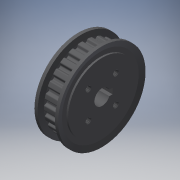
# Autodesk Inventor part: ATP25XL025-A-N8-KC90-QFC20-M3-FC45.0-TPC3_b
Saved by Autodesk Inventor 2017 (Build 210142000, 142)
## iProperties
Category: PARTsolutions
Company: MISUMI
Created: 2017-08-07
Part Number: ATP25XL025-A-N8-KC90-QFC20-M3-FC45.0-TPC3_b
Catalog Web Link: www.cadenas.de
Description: ATP__XL025, ATP__XL031, ATP__ XL037, ATP__XL050, BTP__XL025, BTP__XL031, BTP__XL037, BTP__XL050, KTP__XL025, KTP__XL031, KTP__ XL037, KTP__XL050, NTP__XL025, NTP__XL031, NTP__ XL037, NTP__XL050, MTP__XL025, MTP__ XL037, MTP__XL050, MTPB__XL025, MTPB__ XL037, MTPB__XL050, MTPP__XL025, MTPP__ XL037, MTPP__XL050, STP__XL025, STP__ XL037, STP__XL050_body-Timing Pulleys XL Type
Vendor: MISUMI
Document SubType Name: Modeling
Designer: psAdmin
Manufacturer: MISUMI
Mass: 14.7534 g
Surface Area: 66.1707 cm^2
Volume: 14.7534 cm^3
Density: 1 g/cm^3
Material: 일반
Appearance: PSOLRGB-192-192-192
PSOL_IDENT_0: {$CADENAS_DATA\23d-libs\misumi\metric\51_timing_pulleys\mtp_xl\mtp_xl.prj},737 {VTYP=3D},{NB=ATP25XL
PSOL_IDENT_1: 025-A-N8-KC90-QFC20-M3-FC45.0-TPC3_b},{LINA=ATP25XL025-A-N8-KC90-QFC20-M3-FC45.0-TPC3},{NN=ATP__XL02
PSOL_IDENT_2: 5, ATP__XL031, ATP__ XL037, ATP__XL050, BTP__XL025, BTP__XL031, BTP__XL037, BTP__XL050, KTP__XL025,
PSOL_IDENT_3: KTP__XL031, KTP__ XL037, KTP__XL050, NTP__XL025, NTP__XL031, NTP__ XL037, NTP__XL050, MTP__XL025, MT
PSOL_IDENT_4: P__ XL037, MTP__XL050, MTPB__XL025, MTPB__ XL037, MTPB__XL050, MTPP__XL025, MTPP__ XL037, MTPP__XL05
PSOL_IDENT_5: 0, STP__XL025, STP__ XL037, STP__XL050_body},{DATE=27.04.2017 02:25:46},{GEOMDATE=02.12.2016 00:36:0
PSOL_IDENT_6: 0},{VERSION=},{LINEID=120},{LINESUBID=-1},{WBVAR=MATP,ST,TNW,PS,SBS,DD,Z,J,Q,R,S,T,ALT1,ALT2,M,QSC,Q
PSOL_IDENT_7: FC,QTC,ALT3,K,KSC,KFC,KTC,ALT4,ZM,ZSC,ZFC,ZTC,ALT5,ALT6,ALT7,FC,ALT8,SRG,ALT9,BTC,TL,ALT10,TPC,ALT11
PSOL_IDENT_8: ,BC,ALT12,SLH}  {NB=ATP25XL025-A-N8-KC90-QFC20-M3-FC45.0-TPC3_b},{LINA=ATP25XL025-A-N8-KC90-QFC20-M3
PSOL_IDENT_9: -FC45.0-TPC3},{KT=DUMMY},{PN=ATP25XL025-A-N8-KC90-QFC20-M3-FC45.0-TPC3},{TYPE=ATP},{MATP=A2017},{MAT
PSOL_IDENT_10: PALG= 'A2017','Aluminum Alloy 2000 series','S45C','1045 Carbon Steel Equivalent','SUS304','SUS304' }
PSOL_IDENT_11: ,{ST=CA},{STALG= 'CA','Clear Anodize','BA','Black Anodize','HAT','Hard Clear Anodize','ENP','Electro
PSOL_IDENT_12: less Nickel Plating' },{NT=25},{TNW=XL025},{TNWALG= 'XL025','XL031','XL037','XL050' },{BW=6.4mm (1/4
PSOL_IDENT_13: inch)},{PS=A},{PSALG= 'A','B' },{SBS=N},{SBSALG= 'H','Round Hole','P','Round Hole + Tap','N','New JI
PSOL_IDENT_14: S Keywayed Bore + Tap (Standard)','NK','New JIS Keywayed Bore + Tap (width 4.0mm, height 1.8mm)','C'
PSOL_IDENT_15: ,'Old JIS Keywayed Bore + Tap','V','Stepped Hole','Y','Both Ends Stepped Hole','WB','Double Stepped
PSOL_IDENT_16: Hole' },{DD=8.00},{DDALG=[8:8/1],[10:22/1]},{DDHA=[8:12/1],12.7,[13:31/1]},{DDPA=[8:12/1],12.7,[13:2
PSOL_IDENT_17: 5/1]},{DDNA=[8:8/1],[10:22/1]},{DDNK=[10:10/1]},{DDCA=[10,12,15,16,18,19,20]},{DDVA=[8:12/1],12.7,[1
PSOL_IDENT_18: 3:29/1]},{DDY=[8:29/1]},{DDWB=[8:27/1]},{DDHB=},{DDPB=},{DDNB=},{DDCB=},{DDVFB=},{Z=0},{ZALG=[0]},{Z
PSOL_IDENT_19: MIN=10.000},{ZAMAX=31.000},{ZBMAX=0.000},{DDZ=8.000},{J=0.0},{JALG=[0]},{JMIN=2.000},{JMAX=10},{JPN=
PSOL_IDENT_20: },{Q=0},{QALG=[0]},{QRMIN=10.000},{QRMAX=31},{WBQMIN=12.000},{R=0},{RALG=[0]},{WBRMAX=-2.000},{S=0.0
PSOL_IDENT_21: },{SALG=[0]},{SMAX=6.5},{T=0.0},{TALG=[0]},{TMAX=8},{SBSPN=-N8},{A=7.5},{W=12.5},{L=0},{PD=40.43},{O
PSOL_IDENT_22: D=39.92},{D=0},{DALG=30.000},{DE=35},{F=48},{E=35},{TT=1.6},{BBK=3.000},{TTK=1.4},{ALT1=KC90},{ALT1A
PSOL_IDENT_23: LG= '','w/o KC90 (Set Screw Angle)','KC90','with KC90 (Set Screw Angle)' },{ANG=86.400},{ALT1PN=-KC9
PSOL_IDENT_24: 0},{ALT2=QFC},{ALT2ALG= '','w/o Side Tapped Hole','QFC','with QFC (4 Places Side Tapped Hole)' },{M=
PSOL_IDENT_25: M3},{MALG= 'M3','M4','M5','M6','M8' },{MFTALG= 'M3','M4','M5','M6','M8' },{MSALG='M3','M4','M5','M6'
PSOL_IDENT_26: ,'M8' },{M3D=3.000},{KDML=9.500},{ML=9.500},{MUL=0.500},{PITCH=0.500},{QSC=0.0},{QSCALG=0},{QFC=20.0
PSOL_IDENT_27: },{QFCALG=[15:28/0.5]},{QTC=0.0},{QTCALG=0},{QPCDMIN=15.000},{QPCDMINALG=15.000},{QPCDMAX=28.000},{A
PSOL_IDENT_28: LT2PN=-QFC20-M3},{TAP=6.000},{ALT3=},{ALT3ALG= '','Not applicable' },{K=0.0},{KALG=0},{KMIN=4.000},{
PSOL_IDENT_29: KFTMAX=9.500},{KSMAX=9.000},{KSC=0.0},{KSCALG=0},{KFC=0.0},{KFCALG=0},{KTC=0.0},{KTCALG=0},{KSCMIN=1
PSOL_IDENT_30: 2.000},{KPCDMIN=12.000},{KPCDMAX=31.000},{ALT3PN=},{ALT4=},{ALT4ALG= '','Not applicable' },{ALT4MIN=
PSOL_IDENT_31: 18.500},{ALT4MAX=24.500},{ZM=N/A},{ZMALG= 'N/A' },{ZMFTALG= 'N/A' },{ZMSALG= 'N/A' },{ZMDD1=0.0},{ZM
PSOL_IDENT_32: DD2=0.0},{ZMHH=0.0},{ZSC=0.0},{ZSCALG=[0]},{ZFC=0.0},{ZFCALG=[0]},{ZTC=0.0},{ZTCALG=[0]},{ZPCDMIN=0.
PSOL_IDENT_33: 000},{ZPCDMINALG=0.000},{ZPCDMAX=31.000},{ALT4PN=},{ALT5=},{ALT5ALG= '','w/o Flange not Attached','N
PSOL_IDENT_34: FC','with NFC (Flange not Attached)' },{ALT5PN=},{ALT6=},{ALT6ALG= '','w/o Flange Attached on One Si
PSOL_IDENT_35: de Only','RFC','with RFC (Flange Attached on The Boss Side Only)','LFC','with LFC (Flange Attached o
PSOL_IDENT_36: n The Opposite Side Only)' },{ALT6PN=},{ALT7=FC},{ALT7ALG= '','w/o FC (Flange Cut)','FC','with FC (F
PSOL_IDENT_37: lange Cut)' },{FC=45.0},{FCALG=[41:46/0.5]},{FCMIN=41.0},{FCMAX=46.0},{ALT7PN=-FC45.0},{ALT8=},{ALT8
PSOL_IDENT_38: ALG= '','Not applicable' },{ALT8ALGALG=13.000},{ALT8DD2=0.000},{ALT8MM=0.000},{ALT8NN=0.000},{QC=20.
PSOL_IDENT_39: 000},{KC=0.000},{ZC=0.000},{SRG=0.0},{SRGALG=[0]},{SRGMAX=0.000},{DD2=0.0},{MM=0.00},{NN=0.00},{ALT8
PSOL_IDENT_40: PN=},{ALT9=},{ALT9ALG= '','Not applicable' },{BTC9=9.000},{TL9=1.000},{BTC=0},{BTCALG=[0]},{TL=0.0},
PSOL_IDENT_41: {TLALG=0},{TLMIN=1.000},{TLMAX=-13.000},{BTCL=0},{BTCD=0},{ALT9PN=},{WLBCTL=12.500},{ALT10=TPC},{ALT
PSOL_IDENT_42: 10ALG= '','w/o TPC (Tapped Hole Dimension)','TPC','with TPC (Tapped Hole Dimension)' },{TPC=M3},{TPC
PSOL_IDENT_43: ALG= 'M3','M5' },{TPCM=4.000},{ALT10PN=-TPC3},{ALT11=},{ALT11ALG= '','Not applicable' },{BC=0.0},{BC
PSOL_IDENT_44: ALG=0},{BCMIN=6},{BCMAX=-13},{M1WBC=6.25},{ALT11PN=},{KTT=14.56},{ALT12=},{ALT12ALG= '','w/o SLH (Se
PSOL_IDENT_45: t Screw Length)','SLH','with SLH (Set Screw Length)' },{SLH=0},{SLHALG=[0]},{ALT12PN=},{AC=M3x3},{M1=
PSOL_IDENT_46: 3.000},{M1L=3.000},{KEYA=1.000},{KEYB=0.000},{KEYM=1.000}
NN: 0.00
NT: 25
NB: ATP25XL025-A-N8-KC90-QFC20-M3-FC45.0-TPC3_b
NBSYN: $PN._b
LINA: ATP25XL025-A-N8-KC90-QFC20-M3-FC45.0-TPC3
PN: ATP25XL025-A-N8-KC90-QFC20-M3-FC45.0-TPC3
MATP: Aluminum Alloy 2000 series
ST: Clear Anodize
TNW: XL025
BW: 6.4mm (1/4inch)
PS: A
SBS: New JIS Keywayed Bore + Tap (Standard)
DD: 8.00
Z: 0
J: 0.0
Q: 0
R: 0
S: 0.0
T: 0.0
A: 7.5
W: 12.5
L: 0
PD: 40.43
OD: 39.92
D: 0
F: 48
E: 35
TT: 1.6
ALT1: with KC90 (Set Screw Angle)
ALT2: with QFC (4 Places Side Tapped Hole)
M: M3
QSC: 0.0
QFC: 20.0
QTC: 0.0
ALT3: Not applicable
K: 0.0
KSC: 0.0
KFC: 0.0
KTC: 0.0
ALT4: Not applicable
ZM: N/A
ZMDD1: 0.0
ZMDD2: 0.0
ZMHH: 0.0
ZSC: 0.0
ZFC: 0.0
ZTC: 0.0
ALT5: w/o Flange not Attached
ALT6: w/o Flange Attached on One Side Only
ALT7: with FC (Flange Cut)
FC: 45.0
ALT8: Not applicable
SRG: 0.0
DD2: 0.0
MM: 0.00
ALT9: Not applicable
BTC: 0
TL: 0.0
BTCL: 0
BTCD: 0
ALT10: with TPC (Tapped Hole Dimension)
TPC: M3
ALT11: Not applicable
BC: 0.0
ALT12: w/o SLH (Set Screw Length)
SLH: 0
AC: M3x3
SUPPLIER: MISUMI
ARTICLENO: ATP25XL025-A-N8-KC90-QFC20-M3-FC45.0-TPC3_b
BOMINFO: ATP25XL025-A-N8-KC90-QFC20-M3-FC45.0-TPC3
CREATOR: CADENAS GmbH
Title: ATP25XL025-A-N8-KC90-QFC20-M3-FC45.0-TPC3
Author: Cadenas PARTsolutions
Comments: Timing Pulleys XL Type
Autodesk Inventor part; units mm, degrees
sketch "_____2" plane through (0, 0, 0) normal (0, 0, 1) x (1, 0, 0)
  line L0 (12.5, 0) -> (0, 0)
  line L1 (0, 0) -> (0, 17.5)
  line L2 (0, 17.5) -> (0.9, 17.5)
  line L3 (0.9, 17.5) -> (0.9, 19.749356)
  line L4 (0.9, 19.749356) -> (-0.127996, 23.58589)
  line L5 (-0.127996, 23.58589) -> (1.417485, 24)
  line L6 (1.417485, 24) -> (2.5, 19.96)
  line L7 (2.5, 19.96) -> (10, 19.96)
  line L8 (10, 19.96) -> (11.082515, 24)
  line L9 (11.082515, 24) -> (12.627996, 23.58589)
  line L10 (12.627996, 23.58589) -> (11.6, 19.749356)
  line L11 (11.6, 19.749356) -> (11.6, 17.5)
  line L12 (11.6, 17.5) -> (12.5, 17.5)
  line L13 (12.5, 17.5) -> (12.5, 0)
  line L14 (12.5, 0) -> (0, 0)
  constraints: 30 end point
revolve "Revolution1" add sketch "_____2" angle 360 about axis through (12.5, 0, 0) along (1, 0, 0)
sketch "Sketch2" plane through (12.5, 0, 0) normal (1, 0, 0) x (0, 0, -1)
  point P0 (0, 0)
hole "Hole1" at (12.5, 0, 0) direction (-1, 0, 0) diameter 8 depth 12.5
sketch "_____6" plane through (2.5, 0, 0) normal (1, 0, 0) x (0, 0, -1)
  arc A0 (-19.856937, 3.787913) -> (-20.17511, -1.26931) centre (0, 0) ccw
  arc A1 (-20.17511, -1.26931) -> (-19.225607, -6.246779) centre (0, 0) ccw
  arc A2 (-19.225607, -6.246779) -> (-17.068089, -10.831739) centre (0, 0) ccw
  arc A3 (-17.068089, -10.831739) -> (-13.83812, -14.736101) centre (0, 0) ccw
  arc A4 (-13.83812, -14.736101) -> (-9.738651, -17.71454) centre (0, 0) ccw
  arc A5 (-9.738651, -17.71454) -> (-5.027266, -19.579909) centre (0, 0) ccw
  arc A6 (-5.027266, -19.579909) -> (0, -20.215) centre (0, 0) ccw
  arc A7 (0, -20.215) -> (5.027266, -19.579909) centre (0, 0) ccw
  arc A8 (5.027266, -19.579909) -> (9.738651, -17.71454) centre (0, 0) ccw
  arc A9 (9.738651, -17.71454) -> (13.83812, -14.736101) centre (0, 0) ccw
  arc A10 (13.83812, -14.736101) -> (17.068089, -10.831739) centre (0, 0) ccw
  arc A11 (17.068089, -10.831739) -> (19.225607, -6.246779) centre (0, 0) ccw
  arc A12 (19.225607, -6.246779) -> (20.17511, -1.26931) centre (0, 0) ccw
  arc A13 (20.17511, -1.26931) -> (19.856937, 3.787913) centre (0, 0) ccw
  arc A14 (19.856937, 3.787913) -> (18.291079, 8.607128) centre (0, 0) ccw
  arc A15 (18.291079, 8.607128) -> (15.575925, 12.885526) centre (0, 0) ccw
  arc A16 (15.575925, 12.885526) -> (11.882079, 16.354279) centre (0, 0) ccw
  arc A17 (11.882079, 16.354279) -> (7.441638, 18.795432) centre (0, 0) ccw
  arc A18 (7.441638, 18.795432) -> (2.533611, 20.055599) centre (0, 0) ccw
  arc A19 (2.533611, 20.055599) -> (-2.533611, 20.055599) centre (0, 0) ccw
  arc A20 (-2.533611, 20.055599) -> (-7.441638, 18.795432) centre (0, 0) ccw
  arc A21 (-7.441638, 18.795432) -> (-11.882079, 16.354279) centre (0, 0) ccw
  arc A22 (-11.882079, 16.354279) -> (-15.575925, 12.885526) centre (0, 0) ccw
  arc A23 (-15.575925, 12.885526) -> (-18.291079, 8.607128) centre (0, 0) ccw
  arc A24 (-18.291079, 8.607128) -> (-19.856937, 3.787913) centre (0, 0) ccw
  arc A25 (-19.567688, 0.133077) -> (-19.954959, -0.448576) centre (-19.345113, -0.434867) ccw
  arc A26 (-19.954959, -0.448576) -> (-19.920613, -1.253299) centre (0, 0) ccw
  arc A27 (-19.920613, -1.253299) -> (-19.853829, -2.055981) centre (0, 0) ccw
  arc A28 (-19.853829, -2.055981) -> (-19.396712, -2.58451) centre (-19.247074, -1.993148) ccw
  line L0 (-19.396712, -2.58451) -> (-18.726173, -2.754182)
  arc A29 (-18.275172, -3.239087) -> (-18.726173, -2.754182) centre (-18.875811, -3.345543) ccw
  arc A30 (-18.275172, -3.239087) -> (-18.184213, -3.715914) centre (0, 0) ccw
  arc A31 (-18.425038, -4.332791) -> (-18.184213, -3.715914) centre (-18.781862, -3.838042) ccw
  line L1 (-18.425038, -4.332791) -> (-18.986028, -4.73739)
  arc A32 (-18.986028, -4.73739) -> (-19.216481, -5.397079) centre (-18.629204, -5.232139) ccw
  arc A33 (-19.216481, -5.397079) -> (-18.983088, -6.167979) centre (0, 0) ccw
  arc A34 (-18.983088, -6.167979) -> (-18.718783, -6.928835) centre (0, 0) ccw
  arc A35 (-18.718783, -6.928835) -> (-18.144587, -7.327078) centre (-18.146716, -6.717082) ccw
  line L2 (-18.144587, -7.327078) -> (-17.452919, -7.324664)
  arc A36 (-16.895496, -7.682175) -> (-17.452919, -7.324664) centre (-17.45079, -7.93466) ccw
  arc A37 (-16.895496, -7.682175) -> (-16.688812, -8.121401) centre (0, 0) ccw
  arc A38 (-16.76866, -8.778789) -> (-16.688812, -8.121401) centre (-17.237313, -8.388322) ccw
  line L3 (-16.76866, -8.778789) -> (-17.211406, -9.310189)
  arc A39 (-17.211406, -9.310189) -> (-17.270561, -10.006465) centre (-16.742753, -9.700656) ccw
  arc A40 (-17.270561, -10.006465) -> (-16.852785, -10.695103) centre (0, 0) ccw
  arc A41 (-16.852785, -10.695103) -> (-16.407567, -11.366325) centre (0, 0) ccw
  arc A42 (-16.407567, -11.366325) -> (-15.752371, -11.60926) centre (-15.906133, -11.018957) ccw
  line L4 (-15.752371, -11.60926) -> (-15.083034, -11.434911)
  arc A43 (-14.454214, -11.642565) -> (-15.083034, -11.434911) centre (-14.929271, -12.025213) ccw
  arc A44 (-14.454214, -11.642565) -> (-14.144792, -12.016591) centre (0, 0) ccw
  arc A45 (-14.058646, -12.673183) -> (-14.144792, -12.016591) centre (-14.60968, -12.411533) ccw
  line L5 (-14.058646, -12.673183) -> (-14.355328, -13.297995)
  arc A46 (-14.355328, -13.297995) -> (-14.239468, -13.987107) centre (-13.804294, -13.559645) ccw
  arc A47 (-14.239468, -13.987107) -> (-13.66356, -14.550214) centre (0, 0) ccw
  arc A48 (-13.66356, -14.550214) -> (-13.065403, -15.089627) centre (0, 0) ccw
  arc A49 (-13.065403, -15.089627) -> (-12.370376, -15.161989) centre (-12.66611, -14.628471) ccw
  line L6 (-12.370376, -15.161989) -> (-11.765426, -14.82666)
  arc A50 (-11.10472, -14.871409) -> (-11.765426, -14.82666) centre (-11.469692, -15.360178) ccw
  arc A51 (-11.10472, -14.871409) -> (-10.712003, -15.156734) centre (0, 0) ccw
  arc A52 (-10.465275, -15.771275) -> (-10.712003, -15.156734) centre (-11.064068, -15.654881) ccw
  line L7 (-10.465275, -15.771275) -> (-10.597252, -16.450239)
  arc A53 (-10.597252, -16.450239) -> (-10.313657, -17.088888) centre (-9.99846, -16.566632) ccw
  arc A54 (-10.313657, -17.088888) -> (-9.615803, -17.491081) centre (0, 0) ccw
  arc A55 (-9.615803, -17.491081) -> (-8.902292, -17.864792) centre (0, 0) ccw
  arc A56 (-8.902292, -17.864792) -> (-8.211104, -17.762035) centre (-8.630228, -17.318824) ccw
  line L8 (-8.211104, -17.762035) -> (-7.708553, -17.286796)
  arc A57 (-7.057476, -17.165828) -> (-7.708553, -17.286796) centre (-7.28943, -17.730006) ccw
  arc A58 (-7.057476, -17.165828) -> (-6.606139, -17.344524) centre (0, 0) ccw
  arc A59 (-6.214333, -17.878399) -> (-6.606139, -17.344524) centre (-6.823259, -17.914576) ccw
  line L9 (-6.214333, -17.878399) -> (-6.173312, -18.568854)
  arc A60 (-6.173312, -18.568854) -> (-5.739801, -19.116911) centre (-5.564386, -18.532677) ccw
  arc A61 (-5.739801, -19.116911) -> (-4.96385, -19.33292) centre (0, 0) ccw
  arc A62 (-4.96385, -19.33292) -> (-4.179817, -19.517447) centre (0, 0) ccw
  arc A63 (-4.179817, -19.517447) -> (-3.535899, -19.246026) centre (-4.052077, -18.920972) ccw
  line L10 (-3.535899, -19.246026) -> (-3.167323, -18.660738)
  arc A64 (-2.566784, -18.381654) -> (-3.167323, -18.660738) centre (-2.651145, -18.985793) ccw
  arc A65 (-2.566784, -18.381654) -> (-2.085188, -18.442494) centre (0, 0) ccw
  arc A66 (-1.572921, -18.862158) -> (-2.085188, -18.442494) centre (-2.15372, -19.048632) ccw
  line L11 (-1.572921, -18.862158) -> (-1.36148, -19.520719)
  arc A67 (-1.36148, -19.520719) -> (-0.805292, -19.943749) centre (-0.780681, -19.334245) ccw
  arc A68 (-0.805292, -19.943749) -> (0, -19.96) centre (0, 0) ccw
  arc A69 (0, -19.96) -> (0.805292, -19.943749) centre (0, 0) ccw
  arc A70 (0.805292, -19.943749) -> (1.36148, -19.520719) centre (0.780681, -19.334245) ccw
  line L12 (1.36148, -19.520719) -> (1.572921, -18.862158)
  arc A71 (2.085188, -18.442494) -> (1.572921, -18.862158) centre (2.15372, -19.048632) ccw
  arc A72 (2.085188, -18.442494) -> (2.566784, -18.381654) centre (0, 0) ccw
  arc A73 (3.167323, -18.660738) -> (2.566784, -18.381654) centre (2.651145, -18.985793) ccw
  line L13 (3.167323, -18.660738) -> (3.535899, -19.246026)
  arc A74 (3.535899, -19.246026) -> (4.179817, -19.517447) centre (4.052077, -18.920972) ccw
  arc A75 (4.179817, -19.517447) -> (4.96385, -19.33292) centre (0, 0) ccw
  arc A76 (4.96385, -19.33292) -> (5.739801, -19.116911) centre (0, 0) ccw
  arc A77 (5.739801, -19.116911) -> (6.173312, -18.568854) centre (5.564386, -18.532677) ccw
  line L14 (6.173312, -18.568854) -> (6.214333, -17.878399)
  arc A78 (6.606139, -17.344524) -> (6.214333, -17.878399) centre (6.823259, -17.914576) ccw
  arc A79 (6.606139, -17.344524) -> (7.057476, -17.165828) centre (0, 0) ccw
  arc A80 (7.708553, -17.286796) -> (7.057476, -17.165828) centre (7.28943, -17.730006) ccw
  line L15 (7.708553, -17.286796) -> (8.211104, -17.762035)
  arc A81 (8.211104, -17.762035) -> (8.902292, -17.864792) centre (8.630228, -17.318824) ccw
  arc A82 (8.902292, -17.864792) -> (9.615803, -17.491081) centre (0, 0) ccw
  arc A83 (9.615803, -17.491081) -> (10.313657, -17.088888) centre (0, 0) ccw
  arc A84 (10.313657, -17.088888) -> (10.597252, -16.450239) centre (9.99846, -16.566632) ccw
  line L16 (10.597252, -16.450239) -> (10.465275, -15.771275)
  arc A85 (10.712003, -15.156734) -> (10.465275, -15.771275) centre (11.064068, -15.654881) ccw
  arc A86 (10.712003, -15.156734) -> (11.10472, -14.871409) centre (0, 0) ccw
  arc A87 (11.765426, -14.82666) -> (11.10472, -14.871409) centre (11.469692, -15.360178) ccw
  line L17 (11.765426, -14.82666) -> (12.370376, -15.161989)
  arc A88 (12.370376, -15.161989) -> (13.065403, -15.089627) centre (12.66611, -14.628471) ccw
  arc A89 (13.065403, -15.089627) -> (13.66356, -14.550214) centre (0, 0) ccw
  arc A90 (13.66356, -14.550214) -> (14.239468, -13.987107) centre (0, 0) ccw
  arc A91 (14.239468, -13.987107) -> (14.355328, -13.297995) centre (13.804294, -13.559645) ccw
  line L18 (14.355328, -13.297995) -> (14.058646, -12.673183)
  arc A92 (14.144792, -12.016591) -> (14.058646, -12.673183) centre (14.60968, -12.411533) ccw
  arc A93 (14.144792, -12.016591) -> (14.454214, -11.642565) centre (0, 0) ccw
  arc A94 (15.083034, -11.434911) -> (14.454214, -11.642565) centre (14.929271, -12.025213) ccw
  line L19 (15.083034, -11.434911) -> (15.752371, -11.60926)
  arc A95 (15.752371, -11.60926) -> (16.407567, -11.366325) centre (15.906133, -11.018957) ccw
  arc A96 (16.407567, -11.366325) -> (16.852785, -10.695103) centre (0, 0) ccw
  arc A97 (16.852785, -10.695103) -> (17.270561, -10.006465) centre (0, 0) ccw
  arc A98 (17.270561, -10.006465) -> (17.211406, -9.310189) centre (16.742753, -9.700656) ccw
  line L20 (17.211406, -9.310189) -> (16.76866, -8.778789)
  arc A99 (16.688812, -8.121401) -> (16.76866, -8.778789) centre (17.237313, -8.388322) ccw
  arc A100 (16.688812, -8.121401) -> (16.895496, -7.682175) centre (0, 0) ccw
  arc A101 (17.452919, -7.324664) -> (16.895496, -7.682175) centre (17.45079, -7.93466) ccw
  line L21 (17.452919, -7.324664) -> (18.144587, -7.327078)
  arc A102 (18.144587, -7.327078) -> (18.718783, -6.928835) centre (18.146716, -6.717082) ccw
  arc A103 (18.718783, -6.928835) -> (18.983088, -6.167979) centre (0, 0) ccw
  arc A104 (18.983088, -6.167979) -> (19.216481, -5.397079) centre (0, 0) ccw
  arc A105 (19.216481, -5.397079) -> (18.986028, -4.73739) centre (18.629204, -5.232139) ccw
  line L22 (18.986028, -4.73739) -> (18.425038, -4.332791)
  arc A106 (18.184213, -3.715913) -> (18.425038, -4.332791) centre (18.781862, -3.838042) ccw
  arc A107 (18.184213, -3.715913) -> (18.275172, -3.239087) centre (0, 0) ccw
  arc A108 (18.726173, -2.754182) -> (18.275172, -3.239087) centre (18.875811, -3.345543) ccw
  line L23 (18.726173, -2.754182) -> (19.396712, -2.58451)
  arc A109 (19.396712, -2.58451) -> (19.853829, -2.055981) centre (19.247074, -1.993148) ccw
  arc A110 (19.853829, -2.055981) -> (19.920613, -1.253299) centre (0, 0) ccw
  arc A111 (19.920613, -1.253299) -> (19.954959, -0.448576) centre (0, 0) ccw
  arc A112 (19.954959, -0.448576) -> (19.567688, 0.133077) centre (19.345113, -0.434867) ccw
  line L24 (19.567688, 0.133077) -> (18.923702, 0.385452)
  arc A113 (18.537032, 0.923059) -> (18.923702, 0.385452) centre (19.146277, 0.953396) ccw
  arc A114 (18.537032, 0.923059) -> (18.506552, 1.407526) centre (0, 0) ccw
  arc A115 (18.822793, 1.989356) -> (18.506552, 1.407526) centre (19.114795, 1.453786) ccw
  line L25 (18.822793, 1.989356) -> (19.43007, 2.320454)
  arc A116 (19.43007, 2.320454) -> (19.741387, 2.946058) centre (19.138068, 2.856023) ccw
  arc A117 (19.741387, 2.946058) -> (19.606454, 3.740131) centre (0, 0) ccw
  arc A118 (19.606454, 3.740131) -> (19.439593, 4.528114) centre (0, 0) ccw
  arc A119 (19.439593, 4.528114) -> (18.919838, 4.995182) centre (18.845498, 4.389729) ccw
  line L26 (18.919838, 4.995182) -> (18.233321, 5.079476)
  arc A120 (17.725102, 5.504032) -> (18.233321, 5.079476) centre (18.307662, 5.684929) ccw
  arc A121 (17.725102, 5.504032) -> (17.575097, 5.965698) centre (0, 0) ccw
  arc A122 (17.736708, 6.607895) -> (17.575097, 5.965698) centre (18.152727, 6.161769) ccw
  line L27 (17.736708, 6.607895) -> (18.242565, 7.079614)
  arc A123 (18.242565, 7.079614) -> (18.38852, 7.762985) centre (17.826546, 7.52574) ccw
  arc A124 (18.38852, 7.762985) -> (18.060348, 8.498555) centre (0, 0) ccw
  arc A125 (18.060348, 8.498555) -> (17.702767, 9.220285) centre (0, 0) ccw
  arc A126 (17.702767, 9.220285) -> (17.083185, 9.543422) centre (17.16175, 8.938503) ccw
  line L28 (17.083185, 9.543422) -> (16.397274, 9.454338)
  arc A127 (15.799438, 9.739166) -> (16.397274, 9.454338) centre (16.318709, 10.059257) ccw
  arc A128 (15.799438, 9.739166) -> (15.539335, 10.149024) centre (0, 0) ccw
  arc A129 (15.53616, 10.811236) -> (15.539335, 10.149024) centre (16.050056, 10.482586) ccw
  line L29 (15.53616, 10.811236) -> (15.908813, 11.393936)
  arc A130 (15.908813, 11.393936) -> (15.880235, 12.092136) centre (15.394917, 11.722587) ccw
  arc A131 (15.880235, 12.092136) -> (15.379444, 12.722983) centre (0, 0) ccw
  arc A132 (15.379444, 12.722983) -> (14.85361, 13.333112) centre (0, 0) ccw
  arc A133 (14.85361, 13.333112) -> (14.173133, 13.492013) centre (14.399667, 12.925637) ccw
  line L30 (14.173133, 13.492013) -> (13.530925, 13.235148)
  arc A134 (12.881037, 13.362353) -> (13.530925, 13.235148) centre (13.304391, 13.801525) ccw
  arc A135 (12.881037, 13.362353) -> (12.527178, 13.694649) centre (0, 0) ccw
  arc A136 (12.359418, 14.335267) -> (12.527178, 13.694649) centre (12.938901, 14.144742) ccw
  line L31 (12.359418, 14.335267) -> (12.575451, 14.992336)
  arc A137 (12.575451, 14.992336) -> (12.374136, 15.661493) centre (11.995968, 15.18286) ccw
  arc A138 (12.374136, 15.661493) -> (11.732194, 16.147979) centre (0, 0) ccw
  arc A139 (11.732194, 16.147979) -> (11.071147, 16.60817) centre (0, 0) ccw
  arc A140 (11.071147, 16.60817) -> (10.37253, 16.592852) centre (10.7328, 16.100606) ccw
  line L32 (10.37253, 16.592852) -> (9.814379, 16.184346)
  arc A141 (9.153274, 16.145934) -> (9.814379, 16.184346) centre (9.454109, 16.676592) ccw
  arc A142 (9.153274, 16.145934) -> (8.727893, 16.379789) centre (0, 0) ccw
  arc A143 (8.406088, 16.95856) -> (8.727893, 16.379789) centre (9.014747, 16.918133) ccw
  line L33 (8.406088, 16.95856) -> (8.451928, 17.648712)
  arc A144 (8.451928, 17.648712) -> (8.090525, 18.246781) centre (7.843269, 17.689139) ccw
  arc A145 (8.090525, 18.246781) -> (7.347766, 18.558339) centre (0, 0) ccw
  arc A146 (7.347766, 18.558339) -> (6.593042, 18.839676) centre (0, 0) ccw
  arc A147 (6.593042, 18.839676) -> (5.920184, 18.6511) centre (6.391551, 18.263914) ccw
  line L34 (5.920184, 18.6511) -> (5.481159, 18.116622)
  arc A148 (4.850377, 17.915006) -> (5.481159, 18.116622) centre (5.009791, 18.503807) ccw
  arc A149 (4.850377, 17.915006) -> (4.380202, 18.035726) centre (0, 0) ccw
  arc A150 (3.924573, 18.516285) -> (4.380202, 18.035726) centre (4.524164, 18.628495) ccw
  line L35 (3.924573, 18.516285) -> (3.797339, 19.196154)
  arc A151 (3.797339, 19.196154) -> (3.298556, 19.685556) centre (3.197749, 19.083944) ccw
  arc A152 (3.298556, 19.685556) -> (2.501651, 19.802609) centre (0, 0) ccw
  arc A153 (2.501651, 19.802609) -> (1.700673, 19.887416) centre (0, 0) ccw
  arc A154 (1.700673, 19.887416) -> (1.095851, 19.537431) centre (1.648698, 19.279634) ccw
  line L36 (1.095851, 19.537431) -> (0.803537, 18.910564)
  arc A155 (0.242713, 18.558413) -> (0.803537, 18.910564) centre (0.25069, 19.168361) ccw
  arc A156 (0.242713, 18.558413) -> (-0.242713, 18.558413) centre (0, 0) ccw
  arc A157 (-0.803537, 18.910564) -> (-0.242713, 18.558413) centre (-0.25069, 19.168361) ccw
  line L37 (-0.803537, 18.910564) -> (-1.095851, 19.537431)
  arc A158 (-1.095851, 19.537431) -> (-1.700673, 19.887416) centre (-1.648698, 19.279634) ccw
  arc A159 (-1.700673, 19.887416) -> (-2.501651, 19.802609) centre (0, 0) ccw
  arc A160 (-2.501651, 19.802609) -> (-3.298556, 19.685556) centre (0, 0) ccw
  arc A161 (-3.298556, 19.685556) -> (-3.797339, 19.196154) centre (-3.197749, 19.083944) ccw
  line L38 (-3.797339, 19.196154) -> (-3.924573, 18.516285)
  arc A162 (-4.380202, 18.035726) -> (-3.924573, 18.516285) centre (-4.524164, 18.628495) ccw
  arc A163 (-4.380202, 18.035726) -> (-4.850377, 17.915006) centre (0, 0) ccw
  arc A164 (-5.481159, 18.116622) -> (-4.850377, 17.915006) centre (-5.009791, 18.503807) ccw
  line L39 (-5.481159, 18.116622) -> (-5.920184, 18.6511)
  arc A165 (-5.920184, 18.6511) -> (-6.593042, 18.839676) centre (-6.391551, 18.263914) ccw
  arc A166 (-6.593042, 18.839676) -> (-7.347766, 18.558339) centre (0, 0) ccw
  arc A167 (-7.347766, 18.558339) -> (-8.090524, 18.246781) centre (0, 0) ccw
  arc A168 (-8.090524, 18.246781) -> (-8.451928, 17.648712) centre (-7.843269, 17.689139) ccw
  line L40 (-8.451928, 17.648712) -> (-8.406088, 16.95856)
  arc A169 (-8.727893, 16.379789) -> (-8.406088, 16.95856) centre (-9.014747, 16.918133) ccw
  arc A170 (-8.727893, 16.379789) -> (-9.153274, 16.145934) centre (0, 0) ccw
  arc A171 (-9.814379, 16.184346) -> (-9.153274, 16.145934) centre (-9.454109, 16.676592) ccw
  line L41 (-9.814379, 16.184346) -> (-10.37253, 16.592852)
  arc A172 (-10.37253, 16.592852) -> (-11.071147, 16.60817) centre (-10.7328, 16.100606) ccw
  arc A173 (-11.071147, 16.60817) -> (-11.732194, 16.147979) centre (0, 0) ccw
  arc A174 (-11.732194, 16.147979) -> (-12.374136, 15.661493) centre (0, 0) ccw
  arc A175 (-12.374136, 15.661493) -> (-12.575451, 14.992336) centre (-11.995968, 15.18286) ccw
  line L42 (-12.575451, 14.992336) -> (-12.359418, 14.335267)
  arc A176 (-12.527178, 13.694649) -> (-12.359418, 14.335267) centre (-12.938901, 14.144742) ccw
  arc A177 (-12.527178, 13.694649) -> (-12.881038, 13.362353) centre (0, 0) ccw
  arc A178 (-13.530925, 13.235148) -> (-12.881038, 13.362353) centre (-13.304391, 13.801525) ccw
  line L43 (-13.530925, 13.235148) -> (-14.173133, 13.492013)
  arc A179 (-14.173133, 13.492013) -> (-14.85361, 13.333112) centre (-14.399667, 12.925637) ccw
  arc A180 (-14.85361, 13.333112) -> (-15.379444, 12.722983) centre (0, 0) ccw
  arc A181 (-15.379444, 12.722983) -> (-15.880235, 12.092136) centre (0, 0) ccw
  arc A182 (-15.880235, 12.092136) -> (-15.908813, 11.393936) centre (-15.394917, 11.722587) ccw
  line L44 (-15.908813, 11.393936) -> (-15.53616, 10.811236)
  arc A183 (-15.539335, 10.149024) -> (-15.53616, 10.811236) centre (-16.050056, 10.482586) ccw
  arc A184 (-15.539335, 10.149024) -> (-15.799438, 9.739166) centre (0, 0) ccw
  arc A185 (-16.397274, 9.454338) -> (-15.799438, 9.739166) centre (-16.318709, 10.059257) ccw
  line L45 (-16.397274, 9.454338) -> (-17.083185, 9.543422)
  arc A186 (-17.083185, 9.543422) -> (-17.702767, 9.220285) centre (-17.16175, 8.938503) ccw
  arc A187 (-17.702767, 9.220285) -> (-18.060348, 8.498555) centre (0, 0) ccw
  arc A188 (-18.060348, 8.498555) -> (-18.38852, 7.762985) centre (0, 0) ccw
  arc A189 (-18.38852, 7.762985) -> (-18.242565, 7.079614) centre (-17.826546, 7.52574) ccw
  line L46 (-18.242565, 7.079614) -> (-17.736708, 6.607895)
  arc A190 (-17.575097, 5.965698) -> (-17.736708, 6.607895) centre (-18.152727, 6.161769) ccw
  arc A191 (-17.575097, 5.965698) -> (-17.725102, 5.504031) centre (0, 0) ccw
  arc A192 (-18.233321, 5.079476) -> (-17.725102, 5.504031) centre (-18.307662, 5.684929) ccw
  line L47 (-18.233321, 5.079476) -> (-18.919838, 4.995182)
  arc A193 (-18.919838, 4.995182) -> (-19.439593, 4.528114) centre (-18.845498, 4.389729) ccw
  arc A194 (-19.439593, 4.528114) -> (-19.606454, 3.740131) centre (0, 0) ccw
  arc A195 (-19.606454, 3.740131) -> (-19.741387, 2.946058) centre (0, 0) ccw
  arc A196 (-19.741387, 2.946058) -> (-19.43007, 2.320454) centre (-19.138068, 2.856023) ccw
  line L48 (-19.43007, 2.320454) -> (-18.822793, 1.989356)
  arc A197 (-18.506552, 1.407526) -> (-18.822793, 1.989356) centre (-19.114795, 1.453786) ccw
  arc A198 (-18.506552, 1.407526) -> (-18.537032, 0.923058) centre (0, 0) ccw
  arc A199 (-18.923702, 0.385452) -> (-18.537032, 0.923058) centre (-19.146277, 0.953396) ccw
  line L49 (-18.923702, 0.385452) -> (-19.567688, 0.133077)
  constraints: 400 point on circle, 200 centre point, 100 end point
extrude "Extrusion1" cut sketch "_____6" along normal blind 7.5
sketch "_____43" plane through (0, 0, 0) normal (1, 0, 0) x (0, 0, -1)
  line L0 (-1.5, 5.4) -> (-1.5, 0)
  line L1 (-1.5, 0) -> (1.5, 0)
  line L2 (1.5, 0) -> (1.5, 5.4)
  line L3 (1.5, 5.4) -> (-1.5, 5.4)
  constraints: 8 end point
extrude "Extrusion2" cut sketch "_____43" along normal blind 12.5
sketch "_____14" plane through (0, 0, 0) normal (0, 0, 1) x (1, 0, 0)
  line L0 (500, 0) -> (-500, 0)
  line L1 (-12.5, 48) -> (-12.5, 22.5)
  line L2 (-12.5, 22.5) -> (25, 22.5)
  line L3 (25, 22.5) -> (25, 48)
  line L4 (25, 48) -> (-12.5, 48)
  constraints: 10 end point
revolve "Revolution2" cut sketch "_____14" angle 360 about axis through (500, 0, 0) along (1, 0, 0)
sketch "_____15" plane through (6.25, 0, 0) normal (1, 0, 0) x (0, 0, -1)
  line L0 (0, 0) -> (0, 19.96)
  line L1 (0, 19.96) -> (1.2295, 19.96)
  line L2 (1.2295, 19.96) -> (1.2295, 0)
  line L3 (1.2295, 0) -> (0, 0)
  line L4 (0, 0) -> (0, 19.96)
  constraints: 10 end point
revolve "Revolution3" cut sketch "_____15" angle 360 about axis through (6.25, 0, 0) along (0, -1, 0)
thread "Thread1" size "M3x0.5" class "6H" standard "ISO Metric profile" length 14.56
sketch "_____16" plane through (6.25, 0, 0) normal (1, 0, 0) x (0, 0, -1)
  line L0 (0, 0) -> (19.920613, 1.253299)
  line L1 (19.920613, 1.253299) -> (19.997814, 0.026225)
  line L2 (19.997814, 0.026225) -> (0.077201, -1.227074)
  line L3 (0.077201, -1.227074) -> (0, 0)
  line L4 (0, 0) -> (19.920613, 1.253299)
  constraints: 10 end point
revolve "Revolution4" cut sketch "_____16" angle 360 about axis through (6.25, 0, 0) along (0, -0.0627905, 0.9980267)
thread "Thread2" size "M3x0.5" class "6H" standard "ISO Metric profile" length 15.96
sketch "Sketch8" plane through (12.5, 0, 0) normal (1, 0, 0) x (0, 0, -1)
  point P0 (7.071068, 7.071068)
hole "Hole2" at (12.5, 7.071068, -7.071068) direction (-1, 0, 0) diameter 2.459 depth 8.790148 tip angle 120 countersink diameter 3 countersink angle 90 thread size "M3x0.5" class "6H" standard "ISO Metric profile"
pattern_linear "Rectangular Pattern1" count 2 spacing 14.142136 along (0, 0, 1) count 2 spacing 14.142136 along (0, -1, 0) of "Hole2"
ref_plane "to_screw1_XY" through (6.25, 5.4, 0) normal (0, 1, 0) x (1, 0, 0)
ref_plane "to_screw1_YZ" through (6.25, 5.4, 0) normal (1, 0, 0) x (0, 0, -1)
ref_plane "to_screw1_ZX" through (6.25, 5.4, 0) normal (0, 0, -1) x (0, 1, 0)
ref_plane "to_screw2_XY" through (6.25, 0.251162, -3.992107) normal (0, 0.0627905, -0.9980267) x (1, 0, 0)
ref_plane "to_screw2_YZ" through (6.25, 0.251162, -3.992107) normal (1, 0, 0) x (0, -0.9980267, -0.0627905)
ref_plane "to_screw2_ZX" through (6.25, 0.251162, -3.992107) normal (0, -0.9980267, -0.0627905) x (0, 0.0627905, -0.9980267)
body "Solid1"
